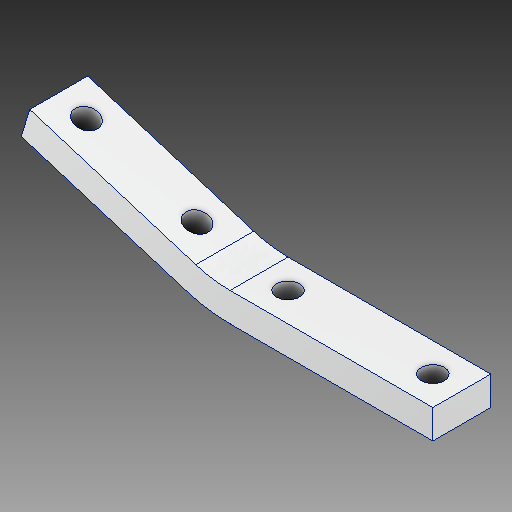
# Autodesk Inventor part: カウンター根本1
Saved by Autodesk Inventor 2020 (Build 240168000, 168)
## iProperties
Created: 2019-07-31
Part Number: カウンター根本1
Material: アルミニウム 6061
Document SubType Name: Modeling
Designer: 雪村
Density: 2.7 g/cm^3
Appearance: アルミニウム - フラット
Mass: 9.00917 g
Surface Area: 24.0363 cm^2
Volume: 3.33673 cm^3
Author: 雪村
Autodesk Inventor part; units mm, degrees
ref_plane "YZ Plane" through (0, 0, 0) normal (1, 0, 0) x (0, 1, 0)
ref_plane "XZ Plane" through (0, 0, 0) normal (0, 1, 0) x (-1, 0, 0)
ref_plane "XY Plane" through (0, 0, 0) normal (0, 0, 1) x (1, 0, 0)
sketch "スケッチ1" plane through (0, 0, 0) normal (0, 0, 1) x (1, 0, 0)
  line L0 (0, 0) -> (-35, 0)
  line L1 (-35, 0) -> (-35, 5)
  line L2 (-35, 5) -> (0, 5)
  line L3 (0, 5) -> (0, 0)
  arc A0 (-42.3998, 1.1202) -> (-35, 0) centre (-35, 25) ccw
  arc A1 (-40.9198, 5.8962) -> (-35, 5) centre (-35, 25) ccw
  line L4 (-40.9198, 5.8962) -> (-42.3998, 1.1202)
  line L5 (-40.9198, 5.8962) -> (-69.5756, 14.776)
  line L6 (-69.5756, 14.776) -> (-71.0555, 10)
  line L7 (-71.0555, 10) -> (-42.3998, 1.1202)
  dimension "d3" = 5
  dimension "d4" = 5
  dimension "d6" = 20
  dimension "d7" = 35
  dimension "d8" = 10
  dimension "d23" = 30
  constraints: 16 end point, 4 point on circle, 2 centre point, 2 horizontal, 2 parallel, 2 tangent, 2 vertical, 1 line through centre, 1 perpendicular, 1 other
  measures "d3" distance of L0.end L1.end
  measures "d4" distance of L4.start L4.end
  measures "d6" radius of A1
  measures "d7" distance of L1.end L2.end
  measures "d8" vertical distance of L6.end L0.start
  measures "d23" distance of L6.end L4.end
extrude "押し出し1" add sketch "スケッチ1" along normal blind 10
sketch "スケッチ2" plane through (-42.3998, 1.1202, 0) normal (-0.295992, -0.9551904, 0) x (0.9551904, -0.295992, 0)
  line L0 (-30, 0) -> (0, 0) projected
  line L1 (0, 0) -> (0, 10) projected
  line L2 (-30, 10) -> (0, 10) projected
  line L3 (-30, 0) -> (-30, 10) projected
  circle A0 centre (-25, 5) radius 2
  circle A1 centre (-5, 5) radius 2
  point P0 (40.8315, 0)
  point P1 (0, 5)
  point P2 (-30, 5)
  dimension "d11" = 4
  dimension "d12" = 4
  dimension "d13" = 5
  dimension "d14" = 5
  constraints: 2 centre point, 2 horizontal alignment, 2 midpoint
  measures "d11" diameter of A0
  measures "d12" diameter of A1
  measures "d13" distance from line of L1 A1.centre
  measures "d14" distance from line of L3 A0.centre
extrude "押し出し2" cut sketch "スケッチ2" against normal through all contours A0 | A1
sketch "スケッチ3" plane through (-35, 0, 0) normal (0, -1, 0) x (1, 0, 0)
  line L0 (0, 0) -> (35, 0) projected
  line L1 (35, 0) -> (35, 10) projected
  line L2 (0, 10) -> (35, 10) projected
  line L3 (0, 0) -> (0, 10) projected
  circle A0 centre (5, 5) radius 2
  circle A1 centre (30, 5) radius 2
  point P0 (35, 5)
  point P1 (0, 5)
  dimension "d17" = 4
  dimension "d18" = 4
  dimension "d19" = 5
  dimension "d20" = 5
  constraints: 2 centre point, 2 horizontal alignment, 2 midpoint
  measures "d17" diameter of A0
  measures "d18" diameter of A1
  measures "d19" distance from line of L1 A1.centre
  measures "d20" distance from line of L3 A0.centre
extrude "押し出し3" cut sketch "スケッチ3" against normal through all contours A0 | A1
